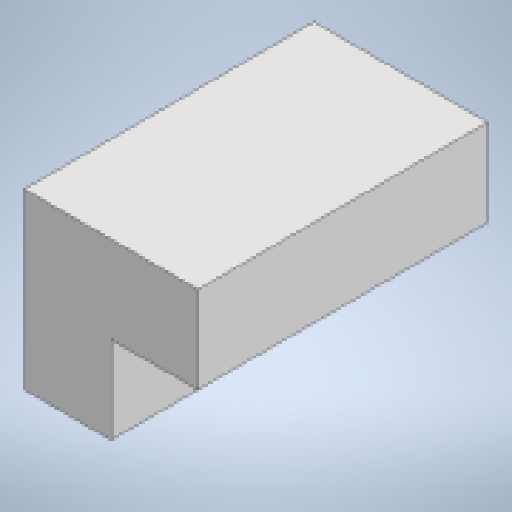
# Autodesk Inventor part: 부품75
Saved by Autodesk Inventor 2024 (Build 280153000, 153)
## iProperties
Created: 2024-09-08
Part Number: 부품75
Material: 일반
Document SubType Name: Modeling
Designer: Eungang
Density: 1 g/cm^3
Appearance: 기본값
Mass: 1.14805 g
Surface Area: 9.67012 cm^2
Volume: 1.14805 cm^3
Author: Eungang
Autodesk Inventor part; units mm, degrees
ref_plane "YZ Plane" through (0, 0, 0) normal (1, 0, 0) x (0, 1, 0)
ref_plane "XZ Plane" through (0, 0, 0) normal (0, 1, 0) x (-1, 0, 0)
ref_plane "XY Plane" through (0, 0, 0) normal (0, 0, 1) x (1, 0, 0)
sketch "스케치1" plane through (0, 0, 0) normal (0, 0, 1) x (1, 0, 0)
  line L0 (0, 0) -> (63.841, 0) projected
  line L1 (63.841, 0) -> (63.841, 6) projected
  line L2 (0, 6) -> (63.841, 6) projected
  line L3 (0, 0) -> (0, 6) projected
  line L4 (46.0408, 0) -> (46.0408, -150) projected
  line L5 (46.0408, -150) -> (51.8408, -150) projected
  line L6 (51.8408, -150) -> (51.8408, 0) projected
  line L7 (51.8408, 0) -> (46.0408, 0) projected
  line L8 (51.8408, 0) -> (63.841, 0)
  line L9 (63.841, 0) -> (63.841, -6)
  line L10 (63.841, -6) -> (51.8408, -6)
  line L11 (51.8408, -6) -> (51.8408, 0)
  line L12 (57.8409, 0) -> (51.8408, 0)
  line L13 (51.8408, 0) -> (51.8408, -12)
  line L14 (51.8408, -12) -> (57.8409, -12)
  line L15 (57.8409, -12) -> (57.8409, 0)
  point P0 (57.8409, -6)
  constraints: 16 end point, 4 parallel, 2 horizontal, 2 perpendicular, 1 midpoint, 1 point on line
extrude "돌출1" add sketch "스케치1" against normal blind 12 contours L0 L15 L10 L6 | L0 L9 L10 L15 | L10 L15 L14 L6
sketch "스케치2" plane through (0, 0, 0) normal (0, 0, 1) x (1, 0, 0)
  line L0 (63.841, -6) -> (57.8409, -6) projected
  line L1 (51.8408, 0) -> (63.841, 0) projected
  line L2 (57.8409, -6) -> (51.8408, -6)
  line L3 (51.8408, -6) -> (51.8408, 0)
  line L4 (51.8408, 0) -> (57.8409, 0)
  line L5 (57.8409, 0) -> (57.8409, -6)
  circle A0 centre (54.8408, -3) radius 1.45
  point P0 (0, 0)
  constraints: 8 end point, 2 parallel, 1 centre point, 1 horizontal, 1 perpendicular
extrude "돌출2" cut sketch "스케치2" against normal up to next contours A0
sketch "스케치3" plane through (57.8409, -6, 0) normal (0, -1, 0) x (1, 0, 0)
  line L0 (6.0001, 0) -> (-6.0001, 0) projected
  line L1 (0, 0) -> (0, -12) projected
  line L2 (6.0001, 0) -> (0, 0)
  line L3 (0, 0) -> (0, -6)
  line L4 (0, -6) -> (6.0001, -6)
  line L5 (6.0001, -6) -> (6.0001, 0)
  circle A0 centre (3.0001, -3) radius 1.35
  point P0 (-57.8409, 0)
  dimension "d6" = 2.7
  constraints: 8 end point, 2 parallel, 1 centre point, 1 horizontal, 1 midpoint, 1 perpendicular
  measures "d6" diameter of A0
extrude "돌출3" cut sketch "스케치3" against normal up to next contours A0
sketch "스케치4" plane through (57.8409, -12, 0) normal (1, 0, 0) x (0, 0, -1)
  line L0 (12, 6) -> (12, 0) projected
  line L1 (0, 6) -> (12, 6) projected
  line L2 (12, 0) -> (6, 0)
  line L3 (6, 0) -> (6, 6)
  line L4 (6, 6) -> (12, 6)
  line L5 (12, 6) -> (12, 0)
  circle A0 centre (9, 3) radius 1.35
  point P0 (0, 12)
  dimension "d9" = 2.7
  constraints: 8 end point, 2 parallel, 1 centre point, 1 horizontal, 1 midpoint, 1 perpendicular
  measures "d9" diameter of A0
extrude "돌출4" cut sketch "스케치4" against normal up to next contours A0
